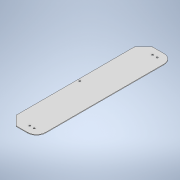
# Autodesk Inventor part: side_ring_guard_piece
Saved by Autodesk Inventor 2022 (Build 260153000, 153)
## iProperties
Created: 2021-12-26
Part Number: side_ring_guard_piece
Material: Generic
Document SubType Name: Modeling
Designer: Alex
Density: 1 g/cm^3
Appearance: Default
Author: Alex
Autodesk Inventor part; units mm, degrees
ref_plane "YZ Plane" through (0, 0, 0) normal (1, 0, 0) x (0, 1, 0)
ref_plane "XZ Plane" through (0, 0, 0) normal (0, 1, 0) x (-1, 0, 0)
ref_plane "XY Plane" through (0, 0, 0) normal (0, 0, 1) x (1, 0, 0)
sketch "Sketch1" plane through (0, 0, 0) normal (0, 1, 0) x (-1, 0, 0)
  line L0 (0, 0) -> (-12.7, 0)
  line L1 (0, 0) -> (12.7, 0)
  line L2 (38.1, 25.4) -> (38.1, 355.6)
  line L3 (12.7, 381) -> (0, 381)
  line L4 (38.1, 355.6) -> (12.7, 381)
  line L5 (38.1, 25.4) -> (12.7, 0)
  circle A0 centre (31.75, 184.15) radius 2.2225
  circle A1 centre (-6.35, 19.05) radius 2.2225
  circle A2 centre (-19.05, 19.05) radius 2.2225
  circle A3 centre (-6.35, 361.95) radius 2.2225
  circle A4 centre (-19.05, 361.95) radius 2.2225
  line L6 (-6.35, 0) -> (0, 0)
  line L7 (0, 381) -> (-19.05, 381)
  line L8 (-44.45, 355.6) -> (-44.45, 25.4)
  line L9 (-19.05, 0) -> (0, 0)
  arc A5 (-19.05, 381) -> (-44.45, 355.6) centre (-19.05, 355.6) ccw
  arc A6 (-44.45, 25.4) -> (-19.05, 0) centre (-19.05, 25.4) ccw
  point P0 (38.1, 381)
  point P1 (38.1, 0)
  point P2 (-44.45, 0)
  point P3 (-44.45, 381)
  dimension "d2" = 38.1
  dimension "d3" = 381
  dimension "d5" = 25.4
  dimension "d6" = 25.4
  dimension "d7" = 25.4
  dimension "d8" = 25.4
  dimension "d12" = 4.445
  dimension "d13" = 4.445
  dimension "d14" = 4.445
  dimension "d15" = 4.445
  dimension "d16" = 4.445
  dimension "d20" = 44.45
  dimension "d21" = 381
  dimension "d22" = 25.4
  constraints: 20 end point, 8 point on line, 7 centre point, 4 point on circle, 4 tangent, 3 horizontal, 2 parallel, 2 perpendicular, 1 equal radius
  measures "d2" distance of L3.end point (38.1, 381)
  measures "d3" distance of point (38.1, 381) point (38.1, 0)
  measures "d5" distance of L2.end point (38.1, 381)
  measures "d6" distance of L3.start point (38.1, 381)
  measures "d7" distance of L2.start point (38.1, 0)
  measures "d8" distance of L1.end point (38.1, 0)
  measures "d12" diameter of A0
  measures "d13" diameter of A1
  measures "d14" diameter of A2
  measures "d15" diameter of A3
  measures "d16" diameter of A4
  measures "d20" distance of L9.end point (-44.45, 0)
  measures "d21" distance of point (-44.45, 0) point (-44.45, 381)
  measures "d22" radius of A5
extrude "Extrusion1" add sketch "Sketch1" along normal blind 1.778
equation "\"d6\" = d5"
equation "\"d7\" = d5"
equation "\"d8\" = d7"
body "Solid1"
